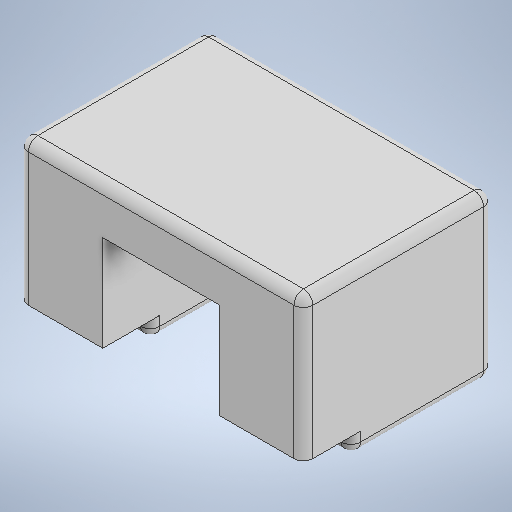
# Autodesk Inventor part: MotorMount
Saved by Autodesk Inventor 2025 (Build 290162000, 162)
## iProperties
Created: 2024-11-13
Part Number: MotorMount
Material: Generic
Document SubType Name: Modeling
Designer: tvoko
Density: 1 g/cm^3
Appearance: Default
Author: tvoko
Autodesk Inventor part; units mm, degrees
ref_plane "YZ Plane" through (0, 0, 0) normal (1, 0, 0) x (0, 1, 0)
ref_plane "XZ Plane" through (0, 0, 0) normal (0, 1, 0) x (-1, 0, 0)
ref_plane "XY Plane" through (0, 0, 0) normal (0, 0, 1) x (1, 0, 0)
sketch "Sketch1" plane through (0, 0, 0) normal (0, 0, 1) x (1, 0, 0)
  line L0 (0, 0) -> (0, 10.1)
  line L1 (0, 10.1) -> (12.3, 10.1)
  line L2 (12.3, 10.1) -> (12.3, 0)
  line L3 (12.3, 0) -> (21.15, 0)
  line L4 (21.15, 0) -> (21.15, 15)
  line L5 (21.15, 15) -> (-8.85, 15)
  line L6 (-8.85, 15) -> (-8.85, 0)
  line L7 (-8.85, 0) -> (0, 0)
  line L8 (6.15, 15) -> (6.15, 10.1) construction
  line L9 (-8.85, 0) -> (0, 0)
  line L10 (0, 0) -> (0, -2)
  line L11 (0, -2) -> (-8.85, -2)
  line L12 (-8.85, -2) -> (-8.85, 0)
  line L13 (12.3, 0) -> (21.15, 0)
  line L14 (21.15, 0) -> (21.15, -2)
  line L15 (21.15, -2) -> (12.3, -2)
  line L16 (12.3, -2) -> (12.3, 0)
  dimension "d0" = 12.3
  dimension "d1" = 30
  dimension "d2" = 15
  dimension "d3" = 10.1
  dimension "d12" = 2
  constraints: 34 end point, 10 perpendicular, 5 parallel, 2 horizontal, 2 midpoint, 1 point on line, 1 vertical
  measures "d0" distance between parallel lines of L0 L2
  measures "d1" distance of L4.end L5.end
  measures "d2" distance of L3.end L4.end
  measures "d3" distance of L1.end L2.end
  measures "d12" distance of L11.end L6.end
extrude "Extrusion1" add sketch "Sketch1" along normal blind 20 contours L7 L6 L5 L4 L3 L2 L1 L0
extrude "Extrusion4" add sketch "Sketch1" along normal blind 15 contours L10 L11 L12 L7 | L3 L14 L15 L16
sketch "Sketch2" plane through (0, 0, 0) normal (0, 0, -1) x (-1, 0, 0)
  line L0 (0, 10.1) -> (-12.3, 10.1) projected
  line L1 (-21.15, 15) -> (8.85, 15) projected
  arc A0 (-9.3, 10.1) -> (-12.3, 7.1) centre (-9.3, 7.1) ccw
  arc A1 (0, 7.1) -> (-3, 10.1) centre (-3, 7.1) ccw
  line L2 (0, 10.1) -> (-12.3, 10.1) projected
  line L3 (0, -2) -> (0, 10.1) projected
  line L4 (8.85, 15) -> (8.85, -2) projected
  line L5 (-21.15, -2) -> (-21.15, 15) projected
  line L6 (-12.3, 10.1) -> (-12.3, -2) projected
  line L7 (0, 0) -> (0, 10.1) projected
  line L8 (8.85, -2) -> (0, -2) projected
  line L9 (-12.3, -2) -> (-21.15, -2) projected
  dimension "d6" = 3
  constraints: 4 point on circle, 4 tangent, 3 point on line, 2 centre point, 1 equal radius
  measures "d6" radius of A0
extrude "Extrusion2" add sketch "Sketch2" against normal blind 10 contours L3 A1 L0 | A0 L6 L0
sketch "Sketch3" plane through (12.3, -2, 0) normal (0, -1, 0) x (1, 0, 0)
  line L0 (8.85, 15) -> (8.85, 20) projected
  line L1 (0, 20) -> (8.85, 20) projected
  line L2 (0, 15) -> (0, 20) projected
  line L3 (-12.3, 15) -> (-12.3, 20) projected
  line L4 (-21.15, 20) -> (-12.3, 20) projected
  line L5 (-21.15, 15) -> (-21.15, 20) projected
  line L6 (4.425, 0) -> (4.425, 20) construction
  line L7 (-16.725, 0) -> (-16.725, 20) construction
  circle A0 centre (4.425, 10) radius 1.5
  circle A1 centre (-16.725, 10) radius 1.5
  line L8 (-21.15, 15) -> (-12.3, 15) projected
  line L9 (0, 15) -> (8.85, 15) projected
  line L10 (0, 0) -> (8.85, 0) projected
  line L11 (8.85, 0) -> (8.85, 15) projected
  line L12 (0, 15) -> (8.85, 15) projected
  line L13 (0, 0) -> (0, 15) projected
  line L14 (-21.15, 0) -> (-12.3, 0) projected
  line L15 (-12.3, 0) -> (-12.3, 15) projected
  line L16 (-21.15, 15) -> (-12.3, 15) projected
  line L17 (-21.15, 0) -> (-21.15, 15) projected
  line L18 (-21.15, 0) -> (-12.3, 0) projected
  dimension "d9" = 3
  constraints: 8 midpoint, 4 end point, 2 centre point, 1 equal radius
  measures "d9" diameter of A0
extrude "Extrusion3" cut sketch "Sketch3" against normal blind 10 contours A0 | A1
fillet "Fillet1" radius 1 21 edges at (15.225, -2, 10) (-5.925, -2, 10) (21.15, -2, 7.5) (16.725, -2, 15) (12.3, -2, 7.5) (16.725, -2, 0) (0, -2, 7.5) (-8.85, -2, 7.5) (-4.425, -2, 15) (0, -1, 15) (-8.85, -1, 15) (-4.425, -2, 0) (21.15, -1, 15) (12.3, -1, 15) (11.4213, 9.2213, 0) (6.15, 10.1, 0) (0.8787, 9.2213, 0) (0, 2.55, 0) (12.3, 2.55, 0) (21.15, 6.5, 0) (-8.85, 6.5, 0)
sketch "Sketch4" plane through (0, 10.1, 20) normal (0, -1, 0) x (1, 0, 0)
  line L0 (9.3, -19) -> (3, -19) projected
  line L1 (9.3, -10) -> (9.3, -19) projected
  line L2 (9.3, -10) -> (12.3, -10) projected
  line L3 (12.3, -10) -> (12.3, 0) projected
  line L4 (0, 0) -> (12.3, 0) projected
  line L5 (0, -10) -> (0, 0) projected
  line L6 (0, -10) -> (3, -10) projected
  line L7 (3, -10) -> (3, -19) projected
  line L8 (12.3, -9) -> (6.3, -9)
  line L9 (6.3, -9) -> (6.3, -7)
  line L10 (6.3, -7) -> (12.3, -7)
  line L11 (12.3, -9.2) -> (9.0739, -9.2) construction
  line L12 (12.3, -6.8) -> (8.8292, -6.8) construction
  point P0 (0, -20)
  dimension "d16" = 1
  dimension "d17" = 2.4
  dimension "d18" = 0.8
  dimension "d19" = 2
  dimension "d20" = 6
  constraints: 10 end point, 4 point on line, 3 horizontal, 2 perpendicular
  measures "d16" distance between parallel lines of L8 L2
  measures "d17" distance between parallel lines of L12 L11
  measures "d18" distance between parallel lines of L11 L2
  measures "d19" distance between parallel lines of L8 L10
  measures "d20" distance of L9.end L10.end
extrude "Extrusion5" add sketch "Sketch4" along normal blind 3 contours L8 L9 L10 L3
chamfer "Chamfer1" distance 2.5 angle 45 1 edges at (6.3, 7.1, 12)
chamfer "Chamfer2" distance 1 angle 45 1 edges at (12.3, 7.1, 12)
fillet "Fillet2" radius 1 11 edges at (6.3, 9.85, 13) (6.3, 9.85, 11) (7.55, 8.35, 11) (7.55, 8.35, 13) (6.3, 9.6, 12) (8.8, 7.1, 12) (10.05, 7.1, 13) (10.05, 7.1, 11) (11.8, 6.6, 11) (11.8, 6.6, 13) (12.3, 6.1, 12)
fillet "Fillet3" radius 0.5 1 edges at (11.4213, 9.2213, 10)
fillet "Fillet4" radius 1 8 edges at (20.8571, 15, 0.2929) (6.15, 15, 0) (-8.5571, 15, 0.2929) (-8.85, 15, 10.5) (6.15, 15, 20) (21.15, 15, 10.5) (21.15, 7.5, 20) (-8.85, 7.5, 20)
body "Solid1"
